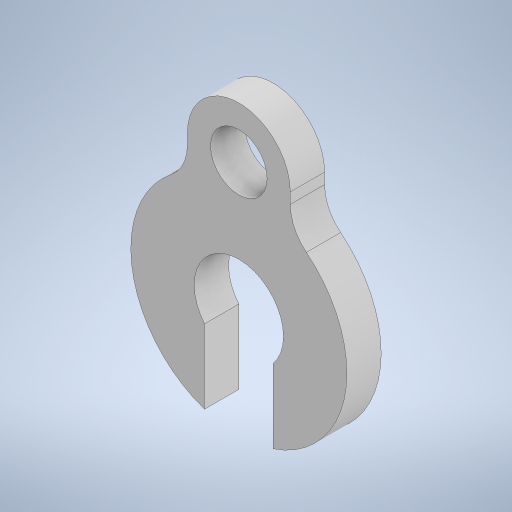
# Autodesk Inventor part: Front Suspension Adjustment Clip
Saved by Autodesk Inventor 2024 (Build 280153000, 153)
## iProperties
Created: 2023-07-07
Part Number: Front Suspension Adjustment Clip
Material: Generic
Document SubType Name: Modeling
Designer: patel
Density: 1 g/cm^3
Appearance: Default
Author: patel
Autodesk Inventor part; units mm, degrees
ref_plane "YZ Plane" through (0, 0, 0) normal (1, 0, 0) x (0, 1, 0)
ref_plane "XZ Plane" through (0, 0, 0) normal (0, 1, 0) x (-1, 0, 0)
ref_plane "XY Plane" through (0, 0, 0) normal (0, 0, 1) x (1, 0, 0)
sketch "Sketch1" plane through (0, 0, 0) normal (0, 0, 1) x (1, 0, 0)
  arc A0 (1.27, -1.0549) -> (-1.27, -1.0549) centre (0, 0) ccw
  circle A1 centre (0, 4.7625) radius 1.0478
  line L0 (-1.27, -1.0549) -> (-1.27, -3.7936)
  line L1 (1.27, -1.0549) -> (1.27, -3.7936)
  line L2 (1.905, 3.5178) -> (1.905, 4.7625)
  line L3 (1.905, 6.8251) -> (-1.905, 6.8251) construction
  line L4 (-1.905, 4.7625) -> (-1.905, 3.5178)
  line L5 (0, -6.1672) -> (0, 8.9905) projected
  arc A2 (1.905, 4.7625) -> (-1.905, 4.7625) centre (0, 4.7625) ccw
  arc A3 (-1.905, 3.5178) -> (-1.27, -3.7936) centre (0, 0) ccw
  arc A4 (1.27, -3.7936) -> (1.905, 3.5178) centre (0, 0) ccw
  point P0 (1.27, -2.4243)
  dimension "d1" = 3.302
  dimension "d2" = 2.0955
  dimension "d3" = 2.54
  dimension "d4" = 4.7625
  dimension "d5" = 3.81
  dimension "d7" = 1.905
  dimension "d8" = 3.81
  dimension "d9" = 1.2447
  dimension "d10" = 4.0005
  dimension "d11" = 4.0005
  dimension "d12" = 1.2447
  constraints: 10 end point, 8 point on circle, 5 centre point, 3 coincident, 2 parallel, 2 vertical, 1 midpoint, 1 point on line
  measures "d1" diameter of A0
  measures "d2" diameter of A1
  measures "d3" distance between parallel lines of L1 L0
  measures "d4" distance of point (0, 0) A1.centre
  measures "d5" distance of L3.end L3.start
  measures "d7" distance from line of point (0, 0) L2
  measures "d8" diameter of A2
  measures "d9" distance of L2.start L2.end
  measures "d10" radius of A3
  measures "d11" radius of A4
  measures "d12" distance of L4.start L4.end
extrude "Extrusion1" add sketch "Sketch1" along normal mid plane 1.27 contours A0 L5 A1 A2 L2 A4 L1 | A0 L0 A3 L4 A2 L5 A1
fillet "Fillet1" radius 1.5875 2 edges at (1.905, 3.5178, 0) (-1.905, 3.5178, 0)
scale "Scale1" factors (10, 10, 10) then translate (0, 0, 5.715) bodies 1
body "Solid1"
